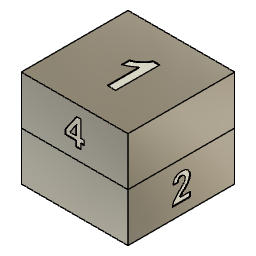
Cubo_Magico v9 (Autodesk Fusion 360 design; units mm, degrees)
Autodesk Fusion 360 part; units mm, degrees
sketch "Boceto1" plane through (0, 0, 0) normal (0, 0, 1) x (1, 0, 0)
  line L0 (27.5, 27.5) -> (-27.5, 27.5)
  line L1 (-27.5, 27.5) -> (-27.5, -27.5)
  line L2 (-27.5, -27.5) -> (27.5, -27.5)
  line L3 (27.5, -27.5) -> (27.5, 27.5)
  line L4 (27.5, 27.5) -> (-27.5, -27.5) construction
  line L5 (-27.5, 27.5) -> (27.5, -27.5) construction
  line L6 (-30.3, -30.3) -> (30.3, -30.3)
  line L7 (30.3, -30.3) -> (30.3, 30.3)
  line L8 (30.3, 30.3) -> (-30.3, 30.3)
  line L9 (-30.3, 30.3) -> (-30.3, -30.3)
  line L10 (-28.9, -28.9) -> (28.9, -28.9)
  line L11 (28.9, -28.9) -> (28.9, 28.9)
  line L12 (28.9, 28.9) -> (-28.9, 28.9)
  line L13 (-28.9, 28.9) -> (-28.9, -28.9)
  line L14 (15.6, 19.5) -> (-15.6, 19.5) construction
  line L15 (-15.6, 19.5) -> (-15.6, -19.5) construction
  line L16 (-15.6, -19.5) -> (15.6, -19.5) construction
  line L17 (15.6, -19.5) -> (15.6, 19.5) construction
  line L18 (15.6, 19.5) -> (-15.6, -19.5) construction
  line L19 (-15.6, 19.5) -> (15.6, -19.5) construction
  line L20 (13.1, 19.5) -> (13.1, 15.9) construction
  circle A0 centre (13.1, 15.9) radius 0.9
  circle A1 centre (13.1, 15.9) radius 2.5
  circle A2 centre (-9.1, -21.864) radius 0.9
  circle A3 centre (-9.1, -21.864) radius 2.5
  line L21 (-8.2867, -19.5) -> (-8.2867, -23) construction
  dimension "d1" = 55
  dimension "d2" = 55
  dimension "d5" = 2.8
  dimension "d13" = 1.4
  dimension "d26" = 31.2
  dimension "d27" = 39
  dimension "d32" = 3.6
  dimension "d33" = 2.5
  dimension "d34" = 1.8
  dimension "d35" = 1.6
  dimension "d38" = 1.8
  dimension "d39" = 1.6
  dimension "d81" = 6.5
  dimension "d82" = 3.5
  constraint horizontal L0
  constraint perpendicular L0 L1
  constraint parallel L0 L2
  constraint parallel L1 L3
  constraint coincident L4 origin
  constraint coincident L5 origin
  constraint horizontal L14
  constraint perpendicular L14 L15
  constraint parallel L14 L16
  constraint parallel L15 L17
  constraint coincident L18 origin
  constraint coincident L19 origin
  constraint coincident L14 L20.start
  constraint perpendicular L14 L20
  constraint coincident L20.end A0.centre
  constraint coincident L16 L21.start
  constraint coincident A3 L21.start
  constraint perpendicular L16 L21
  measures "d1" distance of L1.end L2.end
  measures "d2" distance of L0.end L1.end
  measures "d26" distance of L15.end L16.end
  measures "d27" distance of L14.end L15.end
  measures "d32" distance of L20.start L20.end
  measures "d33" distance of L17 L20
  measures "d34" diameter of A0
  measures "d38" diameter of A2
  measures "d81" distance of L15 A2.centre
  measures "d82" distance of L21.start L21.end
extrude "Extruir1" add sketch "Boceto1" along normal blind 2.8 contours L0 L1 L2 L3 | A0 | A1 | A2 | A3 makes body 1
extrude "Extruir2" add sketch "Boceto1" along normal blind 27.5 contours L6 L7 L8 L9 | L10 L11 L12 L13 bodies 1
ref_plane "PlanoDeObra1" through (0, 0, 27.5) normal (0, 0, 1) x (1, 0, 0)
mirror "Simetría1" about plane through (0, 0, 27.5) normal (0, 0, 1) of bodies 1 makes body 2
extrude "Extruir4" add sketch "Boceto1" against normal blind 18.3333 from surface at 27.5 contours L10 L11 L12 L13 bodies 2
combine "Combinar1" operation cut target body 1 tool bodies 2 keep tools
move_face "CarasDesfase2" offset -0.2 4 faces at (-28.9, 9.6333, 21.3889) (9.6333, 28.9, 21.3889) (28.9, -9.6333, 21.3889) (-9.6333, -28.9, 21.3889) on bodies 1
extrude "Extruir5" add sketch "Boceto1" along normal blind 15 from surface at 2.8 contours A1 | A3 bodies 1
sketch "Boceto3" plane through (0, 30.3, 0) normal (0, 1, 0) x (-1, 0, 0)
  line L0 (9.1, 0) -> (7.6, 0) construction
  line L1 (-13.1, 0) -> (-7.6, 0) construction
  line L2 (-7.6, 0) -> (-7.6, 18) construction
  line L3 (-1.6, 22) -> (-13.6, 22)
  line L4 (-13.6, 22) -> (-13.6, 14)
  line L5 (-13.6, 14) -> (-1.6, 14)
  line L6 (-1.6, 14) -> (-1.6, 22)
  line L7 (-1.6, 22) -> (-13.6, 14) construction
  line L8 (-13.6, 22) -> (-1.6, 14) construction
  line L9 (-30.3, 0) -> (30.3, 0)
  point P0 (9.1, 0)
  point P1 (7.6, 0)
  point P2 (-13.1, 0)
  point P3 (-7.6, 18)
  dimension "d49" = 5.5
  dimension "d50" = 18
  dimension "d51" = 12
  dimension "d52" = 8
  constraint coincident P0 L0.start
  constraint coincident P1 L0.end
  constraint coincident P2 L1.start
  constraint perpendicular L1 L2
  constraint horizontal L3
  constraint perpendicular L3 L4
  constraint parallel L3 L5
  constraint parallel L4 L6
  constraint coincident L7 P3
  constraint coincident L8 P3
  constraint coincident P3 L2.end
  constraint perpendicular L2 L9
  measures "d49" distance of P2 L1.end
  measures "d50" distance of L1.end P3
  measures "d51" distance of L4.end L5.end
  measures "d52" distance of L3.end L4.end
fillet "Empalme3" radius 6 1 edges at (-11.4308, -20.96, 2.8) on bodies 1
fillet "Empalme3" radius 6 1 edges at (10.7692, 16.804, 2.8) on bodies 1
extrude "Extruir6" cut sketch "Boceto3" against normal blind 7 bodies 1
sketch "Boceto4" plane through (30.3, 0, 0) normal (1, 0, 0) x (0, 1, 0)
  line L0 (-30.3, 0) -> (30.3, 0)
  line L1 (30.3, 0) -> (30.3, 27.5)
  line L2 (30.3, 27.5) -> (-30.3, 27.5)
  line L3 (-30.3, 27.5) -> (-30.3, 0)
  line L4 (-30.2971, -0.0064) -> (30.3, 0) construction
  line L5 (30.3, 0) -> (30.2971, 27.5064) construction
  line L6 (30.2971, 27.5064) -> (-30.3, 27.5) construction
  line L7 (-30.3, 27.5) -> (-30.2971, -0.0064) construction
  dimension "d63" = 15
  text T0 "2" font "Arial" height 15 bold align centre middle in box 60.5971 x 27.5064 at (-30.2971, -0.0064) x (1, 0.000105) y (-0.000105, 1) spacing 1 kerned
  constraint coincident L0.end
  constraint coincident L2.end
extrude "Extruir9" cut sketch "Boceto4" against normal blind 0.4 text T0 bodies 1
sketch "Boceto5" plane through (-30.3, 0, 0) normal (-1, 0, 0) x (0, -1, 0)
  line L0 (-30.3, 0) -> (30.3, 0)
  line L1 (30.3, 0) -> (30.3, 27.5)
  line L2 (30.3, 27.5) -> (-30.3, 27.5)
  line L3 (-30.3, 27.5) -> (-30.3, 0)
  line L4 (-30.2971, -0.0064) -> (30.3, 0) construction
  line L5 (30.3, 0) -> (30.2971, 27.5064) construction
  line L6 (30.2971, 27.5064) -> (-30.3, 27.5) construction
  line L7 (-30.3, 27.5) -> (-30.2971, -0.0064) construction
  dimension "d66" = 15
  text T0 "5" font "Arial" height 15 bold align centre middle in box 60.5971 x 27.5064 at (-30.2971, -0.0064) x (1, 0.000105) y (-0.000105, 1) spacing 1 kerned
  constraint coincident L0.end
  constraint coincident L2.end
extrude "Extruir10" cut sketch "Boceto5" against normal blind 0.4 text T0 bodies 1
sketch "Boceto6" plane through (0, 0, 0) normal (0, 0, -1) x (1, 0, 0)
  line L0 (-30.3, -30.3) -> (30.3, -30.3) construction
  line L1 (30.3, -30.3) -> (30.3, 30.3) construction
  line L2 (30.3, 30.3) -> (-30.3, 30.3) construction
  line L3 (-30.3, 30.3) -> (-30.3, -30.3) construction
  point P0 (-30.3, 30.3)
  point P1 (30.3, -30.3)
  dimension "d69" = 25
  text T0 "6" font "Arial" height 25 bold align centre middle in box 60.6 x 60.6 at (-30.3, -30.3) x (1, 0) y (0, 1) spacing 1 kerned
  constraint coincident P1
  constraint coincident P0
extrude "Extruir11" cut sketch "Boceto6" against normal blind 0.4 text T0 bodies 1
sketch "Boceto7" plane through (0, -30.3, 0) normal (0, -1, 0) x (1, 0, 0)
  line L0 (30.3, 55) -> (-30.3, 55)
  line L1 (-30.3, 55) -> (-30.3, 27.5)
  line L2 (-30.3, 27.5) -> (30.3, 27.5)
  line L3 (30.3, 27.5) -> (30.3, 55)
  line L4 (-30.2973, 27.4941) -> (30.3, 27.5) construction
  line L5 (30.3, 27.5) -> (30.2973, 55.0059) construction
  line L6 (30.2973, 55.0059) -> (-30.3, 55) construction
  line L7 (-30.3, 55) -> (-30.2973, 27.4941) construction
  dimension "d72" = 15
  text T0 "4" font "Arial" height 15 bold align centre middle in box 60.5973 x 27.5059 at (-30.2973, 27.4941) x (1, 0.000097) y (-0.000097, 1) spacing 1 kerned
  constraint coincident L2.end
  constraint coincident L0.end
extrude "Extruir12" cut sketch "Boceto7" against normal blind 0.4 text T0 bodies 2
sketch "Boceto8" plane through (0, 0, 55) normal (0, 0, 1) x (-1, 0, 0)
  line L0 (30.3, -30.3) -> (30.3, 30.3)
  line L1 (30.3, 30.3) -> (-30.3, 30.3)
  line L2 (-30.3, 30.3) -> (-30.3, -30.3)
  line L3 (-30.3, -30.3) -> (30.3, -30.3)
  line L4 (30.3, 30.3) -> (-30.3, 30.3) construction
  line L5 (-30.3, 30.3) -> (-30.3, -30.3) construction
  line L6 (-30.3, -30.3) -> (30.3, -30.3) construction
  line L7 (30.3, -30.3) -> (30.3, 30.3) construction
  dimension "d75" = 25
  text T0 "1" font "Arial" height 25 bold align centre middle in box 60.6 x 60.6 at (30.3, 30.3) x (-1, 0) y (0, -1) spacing 1 kerned
  constraint coincident L1.end
  constraint coincident L0.start
extrude "Extruir13" cut sketch "Boceto8" against normal blind 0.4 text T0 bodies 2
sketch "Boceto9" plane through (0, 30.3, 0) normal (0, 1, 0) x (-1, 0, 0)
  line L0 (30.3, 55) -> (-30.3, 55)
  line L1 (-30.3, 55) -> (-30.3, 27.5)
  line L2 (-30.3, 27.5) -> (30.3, 27.5)
  line L3 (30.3, 27.5) -> (30.3, 55)
  line L4 (-30.2973, 27.4941) -> (30.3, 27.5) construction
  line L5 (30.3, 27.5) -> (30.2973, 55.0059) construction
  line L6 (30.2973, 55.0059) -> (-30.3, 55) construction
  line L7 (-30.3, 55) -> (-30.2973, 27.4941) construction
  dimension "d78" = 15
  text T0 "3" font "Arial" height 15 bold align centre middle in box 60.5973 x 27.5059 at (-30.2973, 27.4941) x (1, 0.000097) y (-0.000097, 1) spacing 1 kerned
  constraint coincident L2.end
  constraint coincident L0.end
extrude "Extruir14" cut sketch "Boceto9" against normal blind 0.4 text T0 bodies 2
extrude "Extruir8" cut sketch "Boceto3" against normal blind 9 bodies 2
extrude "Extruir15" cut 1 faces at (-28.4333, -9.1667, 9.1667) along direction (0, 0, 1) blind 13 on bodies 2 bodies 2
equation "d1 = lado"
equation "d2 = lado"
equation "lado = 55 mm"
equation "offset = 2.8 mm"
equation "d5 = offset"
equation "d6 = offset"
equation "d8 = lado / 2"
equation "d10 = lado / 2"
equation "d13 = offset / 2"
equation "d21 = -lado / 3"
equation "d79 = 0 mm - 0.4 mm"
equation "d82 = 6 mm - 2.5 mm"
named bodies: "Base_Cubo", "Tapa_Cubo"
